Autodesk Fusion 360 part; units mm, degrees
(part 2 of 3)
sketch "Sketch29" plane through (1010, 0, 0) normal (1, 0, 0) x (0, 1, 0)
  circle A0 centre (-195, 872.5) radius 13
  circle A1 centre (-195, 872.5) radius 7.5
  line L0 (-180, 857.5) -> (-210, 857.5)
  line L1 (-210, 857.5) -> (-210, 887.5)
  line L2 (-210, 887.5) -> (-180, 887.5)
  line L3 (-180, 887.5) -> (-180, 857.5)
  line L4 (-180, 857.5) -> (-210, 887.5) construction
  line L5 (-210, 857.5) -> (-180, 887.5) construction
  line L6 (-208, 885.5) -> (-182, 885.5)
  line L7 (-182, 885.5) -> (-182, 859.5)
  line L8 (-182, 859.5) -> (-208, 859.5)
  line L9 (-208, 859.5) -> (-208, 885.5)
  point P0 (-195, 872.5)
  dimension "d267" = 30
  dimension "d268" = 2
  dimension "d269" = 2
  dimension "d270" = 2
  constraint horizontal L0
  constraint perpendicular L0 L1
  constraint parallel L0 L2
  constraint parallel L1 L3
  constraint coincident L4 P0
  constraint coincident L5 P0
  constraint coincident P0 A0.centre
  constraint horizontal L6
  constraint vertical L7
  constraint horizontal L8
  constraint vertical L9
  constraint coincident L4 L7.end
  constraint coincident L4 L6.start
  measures "d267" distance of L0.end L1.end
  measures "d268" distance of L2 L6
  measures "d269" distance of L0 L8
  measures "d270" distance of L3 L7
extrude "Extrude17" add sketch "Sketch29" against normal blind 35 contours L0 L1 L2 L3 bodies 9 in component "bin case (1)"
extrude "Extrude18" cut 1 faces at (1023.3333, -530, 856.6667) along direction (0, 1, 0) blind 30 on bodies 9 bodies 9 in component "bin case (1)"
sketch "Sketch30" plane through (1015, 0, 0) normal (-1, 0, 0) x (0, -1, 0)
  line L0 (500, 840) -> (500, 865)
  line L1 (500, 865) -> (180, 865)
  line L2 (180, 865) -> (180, 875)
  line L3 (180, 875) -> (155, 875)
  line L4 (155, 875) -> (155, 825)
  line L5 (155, 825) -> (180, 825)
  line L6 (180, 825) -> (180, 840)
  line L7 (180, 840) -> (500, 840)
extrude "Extrude19" cut 1 faces at (1023.3333, -500, 856.6667) along direction (0, 1, 0) blind 250 on bodies 9 bodies 9 in component "bin case (1)"
sketch "Sketch31" plane through (0, -180, 0) normal (0, -1, 0) x (1, 0, 0)
  line L0 (1010, 887.5) -> (1010, 875)
  line L1 (1010, 875) -> (1015, 875)
  line L2 (1015, 875) -> (1015, 865)
  line L3 (1015, 865) -> (1040, 865)
  line L4 (1040, 865) -> (1040, 900)
  line L5 (1040, 900) -> (-460, 900)
  line L6 (-460, 900) -> (-485, 900)
  line L7 (-485, 900) -> (-485, 875)
  line L8 (-485, 875) -> (-485, 825)
  line L9 (-485, 825) -> (-486, 825)
  line L10 (-486, 825) -> (-519.6212, 807.8463)
  arc A0 (-519.6212, 807.8463) -> (-535, 775.0001) centre (-534.95, 795) ccw
  line L11 (-535, 775.0001) -> (-535, 775)
  line L12 (-535, 775) -> (-534.9999, 775.0001)
  arc A1 (-534.9999, 775.0001) -> (-518.7278, 783.3022) centre (-534.95, 795) ccw
  line L13 (-518.7278, 783.3022) -> (-486, 800)
  line L14 (-486, 800) -> (-485, 800)
  line L15 (-485, 800) -> (-485, 0)
  line L16 (-485, 0) -> (1040, 0)
  line L17 (1040, 0) -> (1040, 800)
  line L18 (1040, 800) -> (1220, 800)
  line L19 (1220, 800) -> (1248.0189, 784.434)
  arc A2 (1248.0189, 784.434) -> (1250.0621, 808.2988) centre (1265, 795) ccw
  line L20 (1250.0621, 808.2988) -> (1220, 825)
  line L21 (1220, 825) -> (1040, 825)
  line L22 (1040, 825) -> (1040, 840)
  line L23 (1040, 840) -> (1015, 840)
  line L24 (1015, 840) -> (1015, 825)
  line L25 (1015, 825) -> (-460, 825)
  line L26 (-460, 825) -> (-460, 875)
  line L27 (-460, 875) -> (975, 875)
  line L28 (975, 875) -> (975, 887.5)
  line L29 (975, 887.5) -> (1010, 887.5)
  line L30 (-460, 800) -> (265, 800)
  line L31 (265, 800) -> (265, 25)
  line L32 (265, 25) -> (-460, 25)
  line L33 (-460, 25) -> (-460, 800)
  line L34 (290, 800) -> (1015, 800)
  line L35 (1015, 800) -> (1015, 25)
  line L36 (1015, 25) -> (290, 25)
  line L37 (290, 25) -> (290, 800)
  line L38 (1040, 900) -> (1015, 900)
  line L39 (1015, 900) -> (1015, 885)
  line L40 (1015, 885) -> (1040, 885)
  line L41 (1040, 885) -> (1040, 900)
  constraint horizontal L38
  constraint vertical L39
  constraint horizontal L40
  constraint vertical L41
  constraint coincident L4.end L5.start
extrude "Extrude20" add sketch "Sketch31" along normal blind 40 contours L4 L5 L38 L39 L40 L41 bodies 9 in component "bin case (1)"
sketch "Sketch32" plane through (0, -220, 0) normal (0, -1, 0) x (1, 0, 0)
  line L0 (1040, 885) -> (1040, 900)
  line L1 (1040, 900) -> (1015, 900)
  line L2 (1015, 900) -> (1015, 885)
  line L3 (1015, 885) -> (1040, 885)
  line L4 (1015, 900) -> (1040, 900)
  line L5 (1040, 900) -> (1040, 875)
  line L6 (1040, 875) -> (1015, 875)
  line L7 (1015, 875) -> (1015, 900)
  dimension "d283" = 25
  constraint horizontal L4
  constraint vertical L5
  constraint horizontal L6
  constraint vertical L7
  constraint coincident L1.end L2.start
  measures "d283" distance of L1.end L6.end
extrude "Extrude21" add sketch "Sketch32" along normal blind 290 bodies 9 in component "bin case (1)"
extrude "Extrude22" cut 1 faces at (1023.3333, -250, 856.6667) along direction (0, 1, 0) blind 10 on bodies 9 bodies 9 in component "bin case (1)"
sketch "Sketch33" plane through (0, 0, 865) normal (0, 0, 1) x (-1, 0, 0)
  line L0 (-1015, 240) -> (-1040, 240)
  line L1 (-1040, 240) -> (-1040, 180)
  line L2 (-1040, 180) -> (-1015, 180)
  line L3 (-1015, 180) -> (-1015, 240)
  line L4 (-1015, 240) -> (-1040, 240)
  line L5 (-1040, 240) -> (-1040, 215)
  line L6 (-1040, 215) -> (-1015, 215)
  line L7 (-1015, 215) -> (-1015, 240)
  constraint horizontal L4
  constraint vertical L5
  constraint horizontal L6
  constraint vertical L7
  constraint coincident L1 L5.end
  constraint coincident L0.start L3.end
extrude "Extrude23" add sketch "Sketch33" along normal blind 20 contours L0 L1 L3 L4 L5 L6 L7 bodies 9 in component "bin case (1)"
sketch "Sketch34" plane through (1015, 0, 0) normal (-1, 0, 0) x (0, -1, 0)
  line L0 (240, 840) -> (240, 875)
  line L1 (240, 875) -> (510, 875)
  line L2 (510, 875) -> (510, 900)
  line L3 (510, 900) -> (180, 900)
  line L4 (180, 900) -> (180, 885)
  line L5 (180, 885) -> (215, 885)
  line L6 (215, 885) -> (215, 865)
  line L7 (215, 865) -> (180, 865)
  line L8 (180, 865) -> (180, 875)
  line L9 (180, 875) -> (155, 875)
  line L10 (155, 875) -> (155, 825)
  line L11 (155, 825) -> (180, 825)
  line L12 (180, 825) -> (180, 840)
  line L13 (180, 840) -> (240, 840)
  circle A0 centre (545, 872.5) radius 27.5
  line L14 (510, 900) -> (545, 882.5)
  line L15 (510, 875) -> (545, 857.5)
  line L16 (545, 857.5) -> (545, 882.5)
  circle A1 centre (545, 872.5) radius 15
  constraint coincident L2.end L3.start
  constraint coincident L1.end L2.start
  constraint parallel L14 L15
  constraint vertical L16
  constraint concentric A0 A1
  constraint coincident L15.end A1
extrude "Extrude24" add sketch "Sketch34" against normal blind 25 contours L2 A0 L14 L15 | A0 L14 L15 A1 | L14 L15 L16 A1 | L15 A1 | L14 L16 A1 picked at (527.3778, 887.7148) bodies 9 in component "bin case (1)"
sketch "Sketch35" plane through (1040, 0, 0) normal (1, 0, 0) x (0, 1, 0)
  line L0 (-240, 875) -> (-240, 840)
  line L1 (-240, 840) -> (-180, 840)
  line L2 (-180, 840) -> (-180, 825)
  line L3 (-180, 825) -> (-155, 825)
  line L4 (-155, 825) -> (-155, 900)
  line L5 (-155, 900) -> (-510, 900)
  line L6 (-510, 900) -> (-538.2297, 885.8852)
  arc A0 (-538.2297, 885.8852) -> (-533, 863.5) centre (-545, 872.5) ccw
  line L7 (-533, 863.5) -> (-510, 875)
  line L8 (-510, 875) -> (-240, 875)
  line L9 (-215, 865) -> (-215, 885)
  line L10 (-215, 885) -> (-180, 885)
  line L11 (-180, 885) -> (-180, 865)
  line L12 (-180, 865) -> (-215, 865)
  circle A1 centre (-545, 872.5) radius 15
  constraint concentric A0 A1
extrude "Extrude25" add sketch "Sketch35" along normal blind 5 contours A0 A1 bodies 9 in component "bin case (1)"
ref_plane "WorkPlane2" through (1245, -360.0396, 862.5) normal (1, 0, 0) x (0, 1, 0)
sketch "Sketch36" plane through (1245, 0, 0) normal (1, 0, 0) x (0, 1, 0)
  circle A0 centre (-545, 872.5) radius 27.5
  circle A1 centre (-195, 872.5) radius 27.5
  circle A2 centre (-545, 872.5) radius 15
  circle A3 centre (-195, 872.5) radius 15
  dimension "d296" = 30
  dimension "d297" = 30
  constraint concentric A0 A2
  constraint concentric A1 A3
  measures "d296" diameter of A2
  measures "d297" diameter of A3
extrude "Extrude6''" add sketch "Sketch36" along normal blind 5 separate body contours A2 | A3 makes body 21 at (1245, -541.6161, 875.3166) makes body 22 at (1245, -199.4126, 875.9009)
copy_body "CutPasteBodies4" bodies 22 21 removing the originals makes body 23 makes body 24 in component "bin case (1)"
sketch "Sketch37" plane through (1250, 0, 0) normal (1, 0, 0) x (0, 1, 0)
  circle A0 centre (-545, 872.5) radius 15
  line L0 (-510.0236, 899.9783) -> (-220.0236, 899.9783)
  line L1 (-220.0236, 899.9783) -> (-220.0236, 874.9783)
  line L2 (-220.0236, 874.9783) -> (-510.0236, 874.9783)
  line L3 (-510.0236, 874.9783) -> (-510.0236, 899.9783)
  line L4 (-510.0236, 874.9783) -> (-545, 857.5)
  line L5 (-510.0236, 899.9783) -> (-545, 882.5)
  line L6 (-545, 882.5) -> (-545, 857.5)
  line L7 (-220.0236, 899.9783) -> (-195, 887.6217)
  line L8 (-220.0236, 874.9783) -> (-195, 862.6217)
  line L9 (-195, 862.6217) -> (-195, 887.6217)
  circle A1 centre (-195, 872.5) radius 15
  circle A2 centre (-195, 872.5) radius 15
  dimension "d300" = 290
  dimension "d301" = 25
  dimension "d302" = 30
  constraint horizontal L0
  constraint vertical L1
  constraint horizontal L2
  constraint vertical L3
  constraint coincident A0 L4.end
  constraint parallel L4 L5
  constraint perpendicular L2 L6
  constraint parallel L7 L8
  constraint perpendicular L2 L9
  constraint coincident L9 A1.centre
  constraint concentric A1 A2
  measures "d300" distance of L0.start L0.end
  measures "d301" distance of L0 L2
  measures "d302" diameter of A1
extrude "Extrude26" add sketch "Sketch37" along normal blind 25 bodies 23 24 in component "bin case (1)"
sketch "Sketch38" plane through (0, 0, 874.9783) normal (0, 0, -1) x (1, 0, 0)
  line L0 (1250, 510.0236) -> (1250, 220.0236)
  line L1 (1250, 220.0236) -> (1275, 220.0236)
  line L2 (1275, 220.0236) -> (1275, 510.0236)
  line L3 (1275, 510.0236) -> (1250, 510.0236)
  line L4 (1250, 220.0236) -> (1275, 220.0236)
  line L5 (1275, 220.0236) -> (1275, 245.0236)
  line L6 (1275, 245.0236) -> (1250, 245.0236)
  line L7 (1250, 245.0236) -> (1250, 220.0236)
  dimension "d305" = 25
  constraint horizontal L4
  constraint vertical L5
  constraint horizontal L6
  constraint vertical L7
  constraint coincident L2 L5.end
  constraint coincident L0.end L1.start
  measures "d305" distance of L4 L6
extrude "Extrude27" add sketch "Sketch38" along normal blind 75 contours L0 L1 L2 L4 L5 L6 L7 bodies 23 in component "bin case (1)"
sketch "Sketch39" plane through (1250, 0, 0) normal (-1, 0, 0) x (0, -1, 0)
  arc A0 (209.7761, 869.9181) -> (195, 887.5) centre (195, 872.5) ccw
  line L0 (209.7761, 869.9181) -> (220.0236, 874.9783)
  line L1 (220.0236, 874.9783) -> (220.0236, 799.9783)
  line L2 (220.0236, 799.9783) -> (245.0236, 799.9783)
  line L3 (245.0236, 799.9783) -> (245.0236, 874.9783)
  line L4 (245.0236, 874.9783) -> (510.0236, 874.9783)
  line L5 (510.0236, 874.9783) -> (533.0041, 863.4946)
  arc A1 (538.2278, 885.8842) -> (533.0041, 863.4946) centre (545, 872.5) ccw
  line L6 (538.2278, 885.8842) -> (510.0236, 899.9783)
  line L7 (510.0236, 899.9783) -> (220.0236, 899.9783)
  line L8 (220.0236, 899.9783) -> (195, 887.6217)
  line L9 (195, 887.6217) -> (195, 887.5)
  line L10 (245.0236, 799.9783) -> (220.0236, 799.9783)
  line L11 (220.0236, 799.9783) -> (220.0236, 824.9783)
  line L12 (220.0236, 824.9783) -> (245.0236, 824.9783)
  line L13 (245.0236, 824.9783) -> (245.0236, 799.9783)
  dimension "d308" = 25
  constraint horizontal L10
  constraint vertical L11
  constraint horizontal L12
  constraint vertical L13
  constraint coincident L2.end L3.start
  measures "d308" distance of L2.end L12.end
extrude "Extrude28" add sketch "Sketch39" along normal blind 235 contours L1 L2 L3 L10 L11 L12 L13 bodies 23 in component "bin case (1)"
sketch "Sketch40" plane through (0, -180, 0) normal (0, -1, 0) x (1, 0, 0)
  line L0 (1015, 885) -> (1015, 900)
  line L1 (1015, 900) -> (-460, 900)
  line L2 (-460, 900) -> (-485, 900)
  line L3 (-485, 900) -> (-485, 875)
  line L4 (-485, 875) -> (-485, 825)
  line L5 (-485, 825) -> (-486, 825)
  line L6 (-486, 825) -> (-519.6212, 807.8463)
  arc A0 (-519.6212, 807.8463) -> (-535, 775.0001) centre (-534.95, 795) ccw
  line L7 (-535, 775.0001) -> (-535, 775)
  line L8 (-535, 775) -> (-534.9999, 775.0001)
  arc A1 (-534.9999, 775.0001) -> (-518.7278, 783.3022) centre (-534.95, 795) ccw
  line L9 (-518.7278, 783.3022) -> (-486, 800)
  line L10 (-486, 800) -> (-485, 800)
  line L11 (-485, 800) -> (-485, 0)
  line L12 (-485, 0) -> (1040, 0)
  line L13 (1040, 0) -> (1040, 800)
  line L14 (1040, 800) -> (1220, 800)
  line L15 (1220, 800) -> (1248.0189, 784.434)
  arc A2 (1248.0189, 784.434) -> (1250.0621, 808.2988) centre (1265, 795) ccw
  line L16 (1250.0621, 808.2988) -> (1220, 825)
  line L17 (1220, 825) -> (1040, 825)
  line L18 (1040, 825) -> (1040, 840)
  line L19 (1040, 840) -> (1015, 840)
  line L20 (1015, 840) -> (1015, 825)
  line L21 (1015, 825) -> (-460, 825)
  line L22 (-460, 825) -> (-460, 875)
  line L23 (-460, 875) -> (975, 875)
  line L24 (975, 875) -> (975, 887.5)
  line L25 (975, 887.5) -> (1010, 887.5)
  line L26 (1010, 887.5) -> (1010, 875)
  line L27 (1010, 875) -> (1015, 875)
  line L28 (1015, 875) -> (1015, 865)
  line L29 (1015, 865) -> (1040, 865)
  line L30 (1040, 865) -> (1040, 885)
  line L31 (1040, 885) -> (1015, 885)
  line L32 (-460, 800) -> (265, 800)
  line L33 (265, 800) -> (265, 25)
  line L34 (265, 25) -> (-460, 25)
  line L35 (-460, 25) -> (-460, 800)
  line L36 (290, 800) -> (1015, 800)
  line L37 (1015, 800) -> (1015, 25)
  line L38 (1015, 25) -> (290, 25)
  line L39 (290, 25) -> (290, 800)
  line L40 (1015, 825) -> (1040, 825)
  line L41 (1040, 825) -> (1040, 800)
  line L42 (1040, 800) -> (1015, 800)
  line L43 (1015, 800) -> (1015, 825)
  constraint horizontal L40
  constraint vertical L41
  constraint horizontal L42
  constraint vertical L43
  constraint coincident L13.end L14.start
  constraint coincident L20.end L21.start
extrude "Extrude29" add sketch "Sketch40" along normal blind 65 contours L40 L41 L42 L43 bodies 9 23 in component "bin case (1)"
sketch "Sketch41" plane through (1015, 0, 0) normal (-1, 0, 0) x (0, -1, 0)
  line L0 (240, 840) -> (240, 875)
  line L1 (240, 875) -> (510, 875)
  line L2 (510, 875) -> (533, 863.5)
  arc A0 (533, 863.5) -> (538.2297, 885.8852) centre (545, 872.5) ccw
  line L3 (538.2297, 885.8852) -> (510, 900)
  line L4 (510, 900) -> (180, 900)
  line L5 (180, 900) -> (180, 885)
  line L6 (180, 885) -> (215, 885)
  line L7 (215, 885) -> (215, 865)
  line L8 (215, 865) -> (180, 865)
  line L9 (180, 865) -> (180, 875)
  line L10 (180, 875) -> (155, 875)
  line L11 (155, 875) -> (155, 825)
  line L12 (155, 825) -> (180, 825)
  line L13 (180, 825) -> (180, 840)
  line L14 (180, 840) -> (240, 840)
sketch "Sketch42" plane through (1015, 0, 0) normal (-1, 0, 0) x (0, -1, 0)
  line L0 (220.0236, 800) -> (220.0236, 799.9783)
  line L1 (220.0236, 799.9783) -> (245.0236, 799.9783)
  line L2 (245.0236, 799.9783) -> (245.0236, 824.9783)
  line L3 (245.0236, 824.9783) -> (245, 824.9783)
  line L4 (245, 824.9783) -> (245, 825)
  line L5 (245, 825) -> (180, 825)
  line L6 (180, 825) -> (180, 800)
  line L7 (180, 800) -> (220.0236, 800)
  line L8 (245.0236, 799.9783) -> (220, 799.9783)
  line L9 (220, 799.9783) -> (220, 825)
  line L10 (220, 825) -> (245.0236, 825)
  line L11 (245.0236, 825) -> (245.0236, 799.9783)
  constraint horizontal L8
  constraint vertical L9
  constraint horizontal L10
  constraint vertical L11
  constraint coincident L5 L9.end
  constraint coincident L1.end L2.start
extrude "Extrude30" add sketch "Sketch42" along normal blind 25 contours L0 L1 L2 L3 L4 L5 L7 L8 L9 L10 L11 bodies 9 in component "bin case (1)"
sketch "Sketch43" plane through (0, 0, 825) normal (0, 0, 1) x (-1, 0, 0)
  line L0 (-1040, 180) -> (-1015, 180)
  line L1 (-1015, 180) -> (-1015, 220)
  line L2 (-1015, 220) -> (-990, 220)
  line L3 (-990, 220) -> (-990, 245)
  line L4 (-990, 245) -> (-1040, 245)
  line L5 (-1040, 245) -> (-1040, 180)
  line L6 (-990, 220) -> (-1015, 220)
  line L7 (-1015, 220) -> (-1015, 245)
  line L8 (-1015, 245) -> (-990, 245)
  line L9 (-990, 245) -> (-990, 220)
  constraint horizontal L6
  constraint vertical L7
  constraint horizontal L8
  constraint vertical L9
  constraint midpoint L4 L7.end
  constraint coincident L2.end L3.start
extrude "Extrude31" add sketch "Sketch43" along normal blind 250 contours L2 L3 L4 L6 L7 L8 L9 bodies 9 in component "bin case (1)"
sketch "Sketch44" plane through (0, -180, 0) normal (0, -1, 0) x (1, 0, 0)
  line L0 (1040, 825) -> (1040, 800)
  line L1 (1040, 800) -> (1220, 800)
  line L2 (1220, 800) -> (1248.0189, 784.434)
  arc A0 (1248.0189, 784.434) -> (1250.0621, 808.2988) centre (1265, 795) ccw
  line L3 (1250.0621, 808.2988) -> (1220, 825)
  line L4 (1220, 825) -> (1040, 825)
  line L5 (1140, 825) -> (1165, 825)
  line L6 (1165, 825) -> (1165, 800)
  line L7 (1165, 800) -> (1140, 800)
  line L8 (1140, 800) -> (1140, 825)
  dimension "d322" = 25
  dimension "d323" = 100
  constraint horizontal L5
  constraint vertical L6
  constraint horizontal L7
  constraint vertical L8
  constraint coincident L1 L6.end
  constraint coincident L4 L5.start
  measures "d322" distance of L6 L8
  measures "d323" distance of L0 L8
extrude "Extrude32" add sketch "Sketch44" along normal blind 45 contours L1 L4 L5 L6 L7 L8 bodies 9 in component "bin case (1)"
sketch "Sketch45" plane through (1015, 0, 0) normal (-1, 0, 0) x (0, -1, 0)
  line L0 (155, 25) -> (180, 25)
  line L1 (180, 25) -> (180, 800)
  line L2 (180, 800) -> (155, 800)
  line L3 (155, 800) -> (155, 25)
  line L4 (220, 800) -> (180, 765)
  line L5 (245, 800) -> (180, 743.125)
  line L6 (180, 765) -> (180, 743.125)
  line L7 (220, 800) -> (245, 800)
  constraint coincident L1 L4.end
  constraint coincident L1 L5.end
  constraint parallel L4 L5
  constraint perpendicular L1 L7
extrude "Extrude33" add sketch "Sketch45" against normal blind 25 contours L1 L4 L5 L6 L7 bodies 9 in component "bin case (1)"
sketch "Sketch46" plane through (0, -245, 0) normal (0, -1, 0) x (1, 0, 0)
  line L0 (990, 824.9783) -> (1040, 824.9783)
  line L1 (1040, 824.9783) -> (1040, 825)
  line L2 (1040, 825) -> (1015, 825)
  line L3 (1015, 825) -> (1015, 875)
  line L4 (1015, 875) -> (1015, 900)
  line L5 (1015, 900) -> (1015, 1075)
  line L6 (1015, 1075) -> (990, 1075)
  line L7 (990, 1075) -> (990, 824.9783)
  line L8 (990, 1075) -> (1015, 1075)
  line L9 (1015, 1075) -> (1015, 1050)
  line L10 (1015, 1050) -> (990, 1050)
  line L11 (990, 1050) -> (990, 1075)
  dimension "d328" = 25
  constraint horizontal L8
  constraint vertical L9
  constraint horizontal L10
  constraint vertical L11
  constraint coincident L6.end L7.start
  measures "d328" distance of L6.end L10.end
extrude "Extrude34" add sketch "Sketch46" along normal blind 200 contours L5 L6 L7 L8 L9 L10 L11 bodies 9 in component "bin case (1)"
sketch "Sketch47" plane through (1015, 0, 0) normal (1, 0, 0) x (0, 1, 0)
  line L0 (-245, 900) -> (-220, 900)
  line L1 (-220, 900) -> (-220, 1075)
  line L2 (-220, 1075) -> (-445, 1075)
  line L3 (-445, 1075) -> (-445, 1050)
  line L4 (-445, 1050) -> (-245, 1050)
  line L5 (-245, 1050) -> (-245, 900)
  line L6 (-445, 1075) -> (-345, 1075)
  line L7 (-345, 1075) -> (-345, 1025)
  line L8 (-345, 1025) -> (-445, 1025)
  line L9 (-445, 1025) -> (-445, 1075)
  dimension "d331" = 50
  constraint horizontal L6
  constraint vertical L7
  constraint horizontal L8
  constraint vertical L9
  constraint coincident L2.end L3.start
  measures "d331" distance of L2.end L8.end
extrude "Extrude1'''''''''" add sketch "Sketch47" along normal blind 250 separate body contours L4 L7 L8 L9 | L2 L3 L4 L6 L7 L9 makes body 25 in component "cam"
sketch "Sketch48" plane through (0, 0, 1025) normal (0, 0, -1) x (1, 0, 0)
  line L0 (1015, 445) -> (1015, 345)
  line L1 (1015, 345) -> (1265, 345)
  line L2 (1265, 345) -> (1265, 445)
  line L3 (1265, 445) -> (1015, 445)
  circle A0 centre (1140, 395) radius 10
  dimension "d336" = 20
  dimension "d337" = 50
  dimension "d338" = 125
  measures "d336" diameter of A0
  measures "d337" distance of L3 A0.centre
  measures "d338" distance of L0 A0.centre
extrude "Extrude2''''''''" add sketch "Sketch48" along normal blind 10 contours A0 bodies 25 in component "cam"
sketch "Sketch49" plane through (0, 0, 1015) normal (0, 0, -1) x (1, 0, 0)
  circle A0 centre (1140, 395) radius 10
  circle A1 centre (1140, 395) radius 5
  constraint concentric A0 A1
extrude "Extrude3''''" add sketch "Sketch49" along normal blind 5 contours A1 bodies 25 in component "cam"
sketch "Sketch50" plane through (0, 0, 900) normal (0, 0, 1) x (-1, 0, 0)
  line L0 (225, 97.8741) -> (185, 155)
  line L1 (185, 155) -> (225, 155)
  line L2 (225, 155) -> (225, 97.8741)
  line L3 (250, 62.1704) -> (250, 155)
  line L4 (250, 155) -> (485, 155)
  line L5 (485, 155) -> (485, 180)
  line L6 (485, 180) -> (460, 180)
  line L7 (460, 180) -> (-1015, 180)
  line L8 (-1015, 180) -> (-1015, 220)
  line L9 (-1015, 220) -> (-1015, 245)
  line L10 (-1015, 245) -> (-1015, 510)
  line L11 (-1015, 510) -> (-1040, 510)
  line L12 (-1040, 510) -> (-1040, 155)
  line L13 (-1040, 155) -> (160, 155)
  line L14 (160, 155) -> (451.3094, -268.9154)
  line L15 (451.3094, -268.9154) -> (471.7882, -254.576)
  line L16 (471.7882, -254.576) -> (250, 62.1704)
  line L17 (-265.0737, 155) -> (-290, 155)
  line L18 (-290, 155) -> (-290, 180)
  line L19 (-290, 180) -> (-265.0737, 180)
  line L20 (-265.0737, 180) -> (-265.0737, 155)
  line L21 (-640, 155) -> (-665, 155)
  line L22 (-665, 155) -> (-665, 180)
  line L23 (-665, 180) -> (-640, 180)
  line L24 (-640, 180) -> (-640, 155)
  line L25 (-1015, 155) -> (-1040, 155)
  line L26 (-1040, 155) -> (-1040, 180)
  line L27 (-1040, 180) -> (-1015, 180)
  line L28 (-1015, 180) -> (-1015, 155)
  constraint horizontal L17
  constraint vertical L18
  constraint horizontal L19
  constraint vertical L20
  constraint coincident L7 L18.end
  constraint coincident L13 L17.start
  constraint horizontal L21
  constraint vertical L22
  constraint horizontal L23
  constraint vertical L24
  constraint coincident L7 L22.end
  constraint coincident L13 L21.start
  constraint horizontal L25
  constraint vertical L26
  constraint horizontal L27
  constraint vertical L28
  constraint coincident L12 L26.end
  constraint coincident L13 L25.start
sketch "Sketch51" plane through (0, -155, 0) normal (0, 1, 0) x (-1, 0, 0)
  line L0 (250, 900) -> (250, 875)
  line L1 (250, 875) -> (460, 875)
  line L2 (460, 875) -> (460, 825)
  line L3 (460, 825) -> (-1015, 825)
  line L4 (-1015, 825) -> (-1015, 875)
  line L5 (-1015, 875) -> (160, 875)
  line L6 (160, 875) -> (160, 900)
  line L7 (160, 900) -> (-1040, 900)
  line L8 (-1040, 900) -> (-1040, 825)
  line L9 (-1040, 825) -> (-1220, 825)
  line L10 (-1220, 825) -> (-1250.0621, 808.2988)
  arc A0 (-1248.0189, 784.434) -> (-1250.0621, 808.2988) centre (-1265, 795) ccw
  line L11 (-1248.0189, 784.434) -> (-1220, 800)
  line L12 (-1220, 800) -> (-1040, 800)
  line L13 (-1040, 800) -> (-1040, 25)
  line L14 (-1040, 25) -> (-1015, 25)
  line L15 (-1015, 25) -> (-1015, 800)
  line L16 (-1015, 800) -> (-290, 800)
  line L17 (-290, 800) -> (-290, 25)
  line L18 (-290, 25) -> (-265, 25)
  line L19 (-265, 25) -> (-265, 800)
  line L20 (-265, 800) -> (460, 800)
  line L21 (460, 800) -> (460, 25)
  line L22 (460, 25) -> (485, 25)
  line L23 (485, 25) -> (485, 800)
  line L24 (485, 800) -> (486, 800)
  line L25 (486, 800) -> (518.7278, 783.3022)
  arc A1 (519.6212, 807.8463) -> (518.7278, 783.3022) centre (534.95, 795) ccw
  line L26 (519.6212, 807.8463) -> (486, 825)
  line L27 (486, 825) -> (485, 825)
  line L28 (485, 825) -> (485, 875)
  line L29 (485, 875) -> (485, 900)
  line L30 (485, 900) -> (250, 900)
  line L31 (-1015, 875) -> (-990, 875)
  line L32 (-990, 875) -> (-990, 900)
  line L33 (-990, 900) -> (-1015, 900)
  line L34 (-1015, 900) -> (-1015, 875)
  line L35 (-615, 875) -> (-640, 875)
  line L36 (-640, 875) -> (-640, 900)
  line L37 (-640, 900) -> (-615, 900)
  line L38 (-615, 900) -> (-615, 875)
  line L39 (-240, 875) -> (-265, 875)
  line L40 (-265, 875) -> (-265, 900)
  line L41 (-265, 900) -> (-240, 900)
  line L42 (-240, 900) -> (-240, 875)
  dimension "d343" = 25
  dimension "d344" = 25
  dimension "d345" = 25
  constraint horizontal L31
  constraint vertical L32
  constraint horizontal L33
  constraint vertical L34
  constraint coincident L7 L32.end
  constraint coincident L4.end L5.start
  constraint horizontal L35
  constraint vertical L36
  constraint horizontal L37
  constraint vertical L38
  constraint coincident L7 L36.end
  constraint coincident L5 L35.start
  constraint horizontal L39
  constraint vertical L40
  constraint horizontal L41
  constraint vertical L42
  constraint coincident L7 L40.end
  constraint coincident L5 L39.start
  measures "d343" distance of L32 L34
  measures "d344" distance of L36 L38
  measures "d345" distance of L40 L42
sketch "Sketch52" plane through (0, 0, 825) normal (0, 0, 1) x (-1, 0, 0)
  line L0 (-1015, 180) -> (-1015, 155)
  line L1 (-1015, 155) -> (460, 155)
  line L2 (460, 155) -> (460, 180)
  line L3 (460, 180) -> (-1015, 180)
  circle A0 centre (-965, 167.5) radius 12.5
  circle A1 centre (-590, 167.5) radius 12.5
  circle A2 centre (-215, 167.5) radius 12.5
  dimension "d346" = 50
  dimension "d349" = 750
  dimension "d350" = 0
  constraint tangent L1 A0
  measures "d346" distance of L0 A0.centre
extrude "Extrude35" add sketch "Sketch52" along normal blind 10 contours A0 | A1 | A2 bodies 9 in component "bin case (1)"
sketch "Sketch53" plane through (0, 0, 835) normal (0, 0, 1) x (-1, 0, 0)
  circle A0 centre (-215, 167.5) radius 12.5
  circle A1 centre (-215, 167.5) radius 17.5
  dimension "d353" = 35
  constraint concentric A0 A1
  measures "d353" diameter of A1
extrude "Extrude1''''''''''" add sketch "Sketch53" along normal blind 40 separate body contours A0 | A1 makes body 26 in component "paddle1"
sketch "Sketch54" plane through (0, 0, 875) normal (0, 0, 1) x (-1, 0, 0)
  circle A0 centre (-215, 167.5) radius 17.5
  circle A1 centre (-215, 167.5) radius 10
  line L0 (-215, 157.5) -> (-215, 177.5)
  line L1 (-215, 177.5) -> (135, 177.5)
  line L2 (135, 177.5) -> (135, 157.5)
  line L3 (135, 157.5) -> (-215, 157.5)
  dimension "d356" = 20
  dimension "d357" = 350
  constraint concentric A0 A1
  constraint perpendicular L0 L1
  constraint parallel L0 L2
  constraint parallel L1 L3
  constraint coincident A1 L0.end
  constraint vertical L0
  constraint coincident A1 L0.start
  measures "d356" diameter of A1
  measures "d357" distance of L0.start L2.end
extrude "Extrude7'" add sketch "Sketch54" against normal blind 40 separate body contours A0 L1 L2 L3 makes body 27
copy_body "CutPasteBodies1''" bodies 27 removing the originals makes body 28 in component "paddle1"
sketch "Sketch55" plane through (0, 0, 825) normal (0, 0, 1) x (-1, 0, 0)
  line L0 (-640.0675, -475) -> (-640.0675, -100)
  line L1 (-640.0675, -100) -> (-290.0675, -100)
  line L2 (-290.0675, -100) -> (-290.0675, -475)
  line L3 (-290.0675, -475) -> (-265.0675, -475)
  line L4 (-265.0675, -475) -> (-265.0675, -100)
  line L5 (-265.0675, -100) -> (84.9325, -100)
  line L6 (84.9325, -100) -> (84.9325, -475)
  line L7 (84.9325, -475) -> (109.9325, -475)
  line L8 (109.9325, -475) -> (109.9325, -100)
  line L9 (109.9325, -100) -> (459.9325, -100)
  line L10 (459.9325, -100) -> (459.9325, -475)
  line L11 (459.9325, -475) -> (484.9325, -475)
  line L12 (484.9325, -475) -> (484.9325, -75)
  line L13 (484.9325, -75) -> (-1220.0675, -75)
  line L14 (-1220.0675, -75) -> (-1220.0675, -100)
  line L15 (-1220.0675, -100) -> (-1040.0675, -100)
  line L16 (-1040.0675, -100) -> (-1040.0675, -475)
  line L17 (-1040.0675, -475) -> (-1015.0675, -475)
  line L18 (-1015.0675, -475) -> (-1015.0675, -100)
  line L19 (-1015.0675, -100) -> (-665.0675, -100)
  line L20 (-665.0675, -100) -> (-665.0675, -475)
  line L21 (-665.0675, -475) -> (-640.0675, -475)
  line L22 (-1005.0675, -110) -> (-675.0675, -110)
  line L23 (-675.0675, -110) -> (-675.0675, -440)
  line L24 (-675.0675, -440) -> (-1005.0675, -440)
  line L25 (-1005.0675, -440) -> (-1005.0675, -110)
  line L26 (-1015.0675, -100) -> (-665.0675, -100)
  line L27 (-665.0675, -100) -> (-665.0675, -450)
  line L28 (-665.0675, -450) -> (-1015.0675, -450)
  line L29 (-1015.0675, -450) -> (-1015.0675, -100)
  dimension "d378" = 10
  dimension "d379" = 10
  dimension "d380" = 10
  dimension "d381" = 330
  dimension "d382" = 10
  constraint horizontal L22
  constraint vertical L23
  constraint horizontal L24
  constraint vertical L25
  constraint horizontal L26
  constraint vertical L27
  constraint horizontal L28
  constraint vertical L29
  constraint coincident L20 L27.end
  constraint coincident L18.end L19.start
  measures "d378" distance of L19 L22
  measures "d379" distance of L20 L23
  measures "d380" distance of L18 L25
  measures "d381" distance of L22 L24
  measures "d382" distance of L24 L28
sketch "Sketch56" plane through (0, 0, 25) normal (0, 0, 1) x (-1, 0, 0)
  line L0 (-665.0675, -350) -> (-665.0675, -450)
  line L1 (-665.0675, -450) -> (-640.0675, -450)
  line L2 (-640.0675, -450) -> (-640.0675, -350)
  line L3 (-640.0675, -350) -> (-290.0675, -350)
  line L4 (-290.0675, -350) -> (-290.0675, -450)
  line L5 (-290.0675, -450) -> (-265.0675, -450)
  line L6 (-265.0675, -450) -> (-265.0675, -350)
  line L7 (-265.0675, -350) -> (84.9325, -350)
  line L8 (84.9325, -350) -> (84.9325, -450)
  line L9 (84.9325, -450) -> (109.9325, -450)
  line L10 (109.9325, -450) -> (109.9325, -350)
  line L11 (109.9325, -350) -> (459.9325, -350)
  line L12 (459.9325, -350) -> (459.9325, -450)
  line L13 (459.9325, -450) -> (484.9325, -450)
  line L14 (484.9325, -450) -> (484.9325, -100)
  line L15 (484.9325, -100) -> (459.9325, -100)
  line L16 (459.9325, -100) -> (459.9325, -200)
  line L17 (459.9325, -200) -> (109.9325, -200)
  line L18 (109.9325, -200) -> (109.9325, -100)
  line L19 (109.9325, -100) -> (84.9325, -100)
  line L20 (84.9325, -100) -> (84.9325, -200)
  line L21 (84.9325, -200) -> (-265.0675, -200)
  line L22 (-265.0675, -200) -> (-265.0675, -100)
  line L23 (-265.0675, -100) -> (-290.0675, -100)
  line L24 (-290.0675, -100) -> (-290.0675, -200)
  line L25 (-290.0675, -200) -> (-640.0675, -200)
  line L26 (-640.0675, -200) -> (-640.0675, -100)
  line L27 (-640.0675, -100) -> (-665.0675, -100)
  line L28 (-665.0675, -100) -> (-665.0675, -200)
  line L29 (-665.0675, -200) -> (-1015.0675, -200)
  line L30 (-1015.0675, -200) -> (-1015.0675, -100)
  line L31 (-1015.0675, -100) -> (-1040.0675, -100)
  line L32 (-1040.0675, -100) -> (-1040.0675, -450)
  line L33 (-1040.0675, -450) -> (-1015.0675, -450)
  line L34 (-1015.0675, -450) -> (-1015.0675, -350)
  line L35 (-1015.0675, -350) -> (-665.0675, -350)
  line L36 (-640.0675, -325) -> (-640.0675, -225)
  line L37 (-640.0675, -225) -> (-290.0675, -225)
  line L38 (-290.0675, -225) -> (-290.0675, -325)
  line L39 (-290.0675, -325) -> (-640.0675, -325)
  line L40 (-665.0675, -325) -> (-1015.0675, -325)
  line L41 (-1015.0675, -325) -> (-1015.0675, -225)
  line L42 (-1015.0675, -225) -> (-665.0675, -225)
  line L43 (-665.0675, -225) -> (-665.0675, -325)
  line L44 (109.9325, -325) -> (109.9325, -225)
  line L45 (109.9325, -225) -> (459.9325, -225)
  line L46 (459.9325, -225) -> (459.9325, -325)
  line L47 (459.9325, -325) -> (109.9325, -325)
  line L48 (84.9325, -325) -> (-265.0675, -325)
  line L49 (-265.0675, -325) -> (-265.0675, -225)
  line L50 (-265.0675, -225) -> (84.9325, -225)
  line L51 (84.9325, -225) -> (84.9325, -325)
  line L52 (-995.0675, -120) -> (-685.0675, -120)
  line L53 (-685.0675, -120) -> (-685.0675, -430)
  line L54 (-685.0675, -430) -> (-995.0675, -430)
  line L55 (-995.0675, -430) -> (-995.0675, -120)
  line L56 (-1015.0675, -100) -> (-665.0675, -100)
  line L57 (-665.0675, -450) -> (-1015.0675, -450)
  line L58 (-665.0675, -100) -> (-665.0675, -450)
  line L59 (-1015.0675, -450) -> (-1015.0675, -100)
  dimension "d383" = 20
  dimension "d384" = 20
  dimension "d385" = 20
  dimension "d386" = 20
  constraint horizontal L52
  constraint vertical L53
  constraint horizontal L54
  constraint vertical L55
  measures "d383" distance of L52 L56
  measures "d384" distance of L54 L57
  measures "d385" distance of L53 L58
  measures "d386" distance of L55 L59
loft "Loft1" add profiles "Sketch55", "Sketch56" section 1 contours L18 L19 L20 L26 L27 L28 L29 | L22 L23 L24 L25 section 2 contours L35 L53 L54 L55 | L35 L40 L53 L55 | L40 L42 L53 L55 | L29 L42 L53 L55 | L29 L52 L53 L55 separate body makes body 29 in component "bin"
shell "Shell1" thickness 10 removed faces 1 at (781.7342, 216.6667, 825) on bodies 29 in component "bin"
loft "Loft1'" add profiles "Sketch55", "Sketch56" section 1 contours L18 L19 L20 L26 L27 L28 L29 | L22 L23 L24 L25 section 2 contours L35 L53 L54 L55 | L35 L40 L53 L55 | L40 L42 L53 L55 | L29 L42 L53 L55 | L29 L52 L53 L55 separate body makes body 30 in component "bin (1)"
shell "Shell1'" thickness 10 removed faces 1 at (781.7342, 216.6667, 825) on bodies 30 in component "bin (1)"
loft "Loft1''" add profiles "Sketch55", "Sketch56" section 1 contours L18 L19 L20 L26 L27 L28 L29 | L22 L23 L24 L25 section 2 contours L35 L53 L54 L55 | L35 L40 L53 L55 | L40 L42 L53 L55 | L29 L42 L53 L55 | L29 L52 L53 L55 separate body makes body 31 in component "bin (2)"
shell "Shell1''" thickness 10 removed faces 1 at (781.7342, 216.6667, 825) on bodies 31 in component "bin (2)"
loft "Loft1'''" add profiles "Sketch55", "Sketch56" section 1 contours L18 L19 L20 L26 L27 L28 L29 | L22 L23 L24 L25 section 2 contours L35 L53 L54 L55 | L35 L40 L53 L55 | L40 L42 L53 L55 | L29 L42 L53 L55 | L29 L52 L53 L55 separate body makes body 32 in component "bin (3)"
shell "Shell1'''" thickness 10 removed faces 1 at (781.7342, 216.6667, 825) on bodies 32 in component "bin (3)"
sketch "Sketch57" plane through (-484.9325, 0, 0) normal (-1, 0, 0) x (0, -1, 0)
  line L0 (-100, 0) -> (-100, 25)
  line L1 (-100, 25) -> (-450, 25)
  line L2 (-450, 25) -> (-450, 800)
  line L3 (-450, 800) -> (-100, 800)
  line L4 (-100, 800) -> (-100, 25)
  line L5 (-100, 25) -> (-75, 25)
  line L6 (-75, 25) -> (-75, 825)
  line L7 (-75, 825) -> (-475, 825)
  line L8 (-475, 825) -> (-475, 0)
  line L9 (-475, 0) -> (-100, 0)
  line L10 (-450, 75) -> (-475, 75)
  line L11 (-475, 75) -> (-475, 100)
  line L12 (-475, 100) -> (-450, 100)
  line L13 (-450, 100) -> (-450, 75)
  dimension "d388" = 25
  dimension "d389" = 50
  constraint horizontal L10
  constraint vertical L11
  constraint horizontal L12
  constraint vertical L13
  constraint coincident L8 L11.end
  constraint coincident L2 L10.start
  measures "d388" distance of L10 L12
  measures "d389" distance of L1 L10
extrude "Extrude36" add sketch "Sketch57" against normal blind 1500 contours L2 L8 L10 L11 L12 L13 bodies 9 in component "bin case (1)"
sketch "Sketch58" plane through (0, 475, 0) normal (0, 1, 0) x (-1, 0, 0)
  line L0 (-1015.0675, 100) -> (-1015.0675, 825)
  line L1 (-1015.0675, 825) -> (-1040.0675, 825)
  line L2 (-1040.0675, 825) -> (-1040.0675, 0)
  line L3 (-1040.0675, 0) -> (484.9325, 0)
  line L4 (484.9325, 0) -> (484.9325, 825)
  line L5 (484.9325, 825) -> (459.9325, 825)
  line L6 (459.9325, 825) -> (459.9325, 100)
  line L7 (459.9325, 100) -> (109.9325, 100)
  line L8 (109.9325, 100) -> (109.9325, 825)
  line L9 (109.9325, 825) -> (84.9325, 825)
  line L10 (84.9325, 825) -> (84.9325, 100)
  line L11 (84.9325, 100) -> (-265.0675, 100)
  line L12 (-265.0675, 100) -> (-265.0675, 825)
  line L13 (-265.0675, 825) -> (-290.0675, 825)
  line L14 (-290.0675, 825) -> (-290.0675, 100)
  line L15 (-290.0675, 100) -> (-640.0675, 100)
  line L16 (-640.0675, 100) -> (-640.0675, 825)
  line L17 (-640.0675, 825) -> (-665.0675, 825)
  line L18 (-665.0675, 825) -> (-665.0675, 100)
  line L19 (-665.0675, 100) -> (-1015.0675, 100)
  line L20 (459.9325, 75) -> (459.9325, 25)
  line L21 (459.9325, 25) -> (109.9325, 25)
  line L22 (109.9325, 25) -> (109.9325, 75)
  line L23 (109.9325, 75) -> (459.9325, 75)
  line L24 (-1015.0675, 75) -> (-665.0675, 75)
  line L25 (-665.0675, 75) -> (-665.0675, 25)
  line L26 (-665.0675, 25) -> (-1015.0675, 25)
  line L27 (-1015.0675, 25) -> (-1015.0675, 75)
  line L28 (-290.0675, 75) -> (-290.0675, 25)
  line L29 (-290.0675, 25) -> (-640.0675, 25)
  line L30 (-640.0675, 25) -> (-640.0675, 75)
  line L31 (-640.0675, 75) -> (-290.0675, 75)
  line L32 (-265.0675, 75) -> (84.9325, 75)
  line L33 (84.9325, 75) -> (84.9325, 25)
  line L34 (84.9325, 25) -> (-265.0675, 25)
  line L35 (-265.0675, 25) -> (-265.0675, 75)
  line L36 (-1015.0675, 75) -> (-1040.0675, 75)
  line L37 (-1040.0675, 75) -> (-1040.0675, 100)
  line L38 (-1040.0675, 100) -> (-1015.0675, 100)
  line L39 (-1015.0675, 100) -> (-1015.0675, 75)
  line L40 (-665.0675, 100) -> (-640.0675, 100)
  line L41 (-640.0675, 100) -> (-640.0675, 75)
  line L42 (-640.0675, 75) -> (-665.0675, 75)
  line L43 (-665.0675, 75) -> (-665.0675, 100)
  line L44 (-290.0675, 100) -> (-265.0675, 100)
  line L45 (-265.0675, 100) -> (-265.0675, 75)
  line L46 (-265.0675, 75) -> (-290.0675, 75)
  line L47 (-290.0675, 75) -> (-290.0675, 100)
  line L48 (84.9325, 100) -> (109.9325, 100)
  line L49 (109.9325, 100) -> (109.9325, 75)
  line L50 (109.9325, 75) -> (84.9325, 75)
  line L51 (84.9325, 75) -> (84.9325, 100)
  line L52 (459.9325, 100) -> (484.9325, 100)
  line L53 (484.9325, 100) -> (484.9325, 75)
  line L54 (484.9325, 75) -> (459.9325, 75)
  line L55 (459.9325, 75) -> (459.9325, 100)
  dimension "d394" = 1500
  dimension "d395" = 0
  constraint horizontal L36
  constraint vertical L37
  constraint horizontal L38
  constraint vertical L39
  constraint coincident L2 L37.end
  constraint coincident L24.start L27.end
extrude "Extrude37" add sketch "Sketch58" against normal blind 400 contours L2 L36 L37 L38 L39 | L40 L41 L42 L43 | L44 L45 L46 L47 | L48 L49 L50 L51 | L4 L52 L53 L54 L55 bodies 9 in component "bin case (1)"
sketch "Sketch59" plane through (-484.9325, 0, 0) normal (-1, 0, 0) x (0, -1, 0)
  line L0 (-450, 100) -> (-450, 800)
  line L1 (-450, 800) -> (-100, 800)
  line L2 (-100, 800) -> (-100, 100)
  line L3 (-100, 100) -> (-450, 100)
  line L4 (-450, 75) -> (-100, 75)
  line L5 (-100, 75) -> (-100, 25)
  line L6 (-100, 25) -> (-75, 25)
  line L7 (-75, 25) -> (-75, 825)
  line L8 (-75, 825) -> (-475, 825)
  line L9 (-475, 825) -> (-475, 0)
  line L10 (-475, 0) -> (-100, 0)
  line L11 (-100, 0) -> (-100, 25)
  line L12 (-100, 25) -> (-450, 25)
  line L13 (-450, 25) -> (-450, 75)
  line L14 (-100, 100) -> (-75, 100)
  line L15 (-75, 100) -> (-75, 75)
  line L16 (-75, 75) -> (-100, 75)
  line L17 (-100, 75) -> (-100, 100)
  constraint horizontal L14
  constraint vertical L15
  constraint horizontal L16
  constraint vertical L17
  constraint coincident L7 L15.end
  constraint coincident L2.end L3.start
extrude "Extrude38" add sketch "Sketch59" against normal blind 1525 contours L7 L14 L15 L16 L17 bodies 9 in component "bin case (1)"
extrude "Extrude39" cut 1 faces at (998.3333, -445, 1066.6667) along direction (0, 1, 0) blind 25 on bodies 9 bodies 9 in component "bin case (1)"
sketch "Sketch60" plane through (0, 0, 825) normal (0, 0, 1) x (-1, 0, 0)
  line L0 (-640.0675, -475) -> (-640.0675, -100)
  line L1 (-640.0675, -100) -> (-290.0675, -100)
  line L2 (-290.0675, -100) -> (-290.0675, -475)
  line L3 (-290.0675, -475) -> (-265.0675, -475)
  line L4 (-265.0675, -475) -> (-265.0675, -100)
  line L5 (-265.0675, -100) -> (84.9325, -100)
  line L6 (84.9325, -100) -> (84.9325, -475)
  line L7 (84.9325, -475) -> (109.9325, -475)
  line L8 (109.9325, -475) -> (109.9325, -100)
  line L9 (109.9325, -100) -> (459.9325, -100)
  line L10 (459.9325, -100) -> (459.9325, -475)
  line L11 (459.9325, -475) -> (484.9325, -475)
  line L12 (484.9325, -475) -> (484.9325, -75)
  line L13 (484.9325, -75) -> (-1220.0675, -75)
  line L14 (-1220.0675, -75) -> (-1220.0675, -100)
  line L15 (-1220.0675, -100) -> (-1040.0675, -100)
  line L16 (-1040.0675, -100) -> (-1040.0675, -475)
  line L17 (-1040.0675, -475) -> (-1015.0675, -475)
  line L18 (-1015.0675, -475) -> (-1015.0675, -100)
  line L19 (-1015.0675, -100) -> (-665.0675, -100)
  line L20 (-665.0675, -100) -> (-665.0675, -475)
  line L21 (-665.0675, -475) -> (-640.0675, -475)
  line L22 (-1220.0675, -75) -> (-1040.0675, -75)
  line L23 (-1040.0675, -75) -> (-1040.0675, -87.5)
  line L24 (-1040.0675, -87.5) -> (-1220.0675, -87.5)
  line L25 (-1220.0675, -87.5) -> (-1220.0675, -75)
  dimension "d406" = 180
  constraint horizontal L22
  constraint vertical L23
  constraint horizontal L24
  constraint vertical L25
  constraint coincident L13.end L14.start
  measures "d406" distance of L23 L25
extrude "Extrude1'''''''''''" add sketch "Sketch60" along normal blind 150 separate body contours L13 L14 L22 L23 L24 L25 makes body 33 in component "limit"
extrude "Extrude2'''''''''" add 1 faces at (1220.0675, 79.1667, 875) along direction (1, 0, 0) blind 50 on bodies 33 bodies 33 in component "limit"
sketch "Sketch61" plane through (0, 0, 825) normal (0, 0, 1) x (-1, 0, 0)
  line L0 (-640.0675, -475) -> (-640.0675, -100)
  line L1 (-640.0675, -100) -> (-290.0675, -100)
  line L2 (-290.0675, -100) -> (-290.0675, -475)
  line L3 (-290.0675, -475) -> (-265.0675, -475)
  line L4 (-265.0675, -475) -> (-265.0675, -100)
  line L5 (-265.0675, -100) -> (84.9325, -100)
  line L6 (84.9325, -100) -> (84.9325, -475)
  line L7 (84.9325, -475) -> (109.9325, -475)
  line L8 (109.9325, -475) -> (109.9325, -100)
  line L9 (109.9325, -100) -> (459.9325, -100)
  line L10 (459.9325, -100) -> (459.9325, -475)
  line L11 (459.9325, -475) -> (484.9325, -475)
  line L12 (484.9325, -475) -> (484.9325, -75)
  line L13 (484.9325, -75) -> (-1220.0675, -75)
  line L14 (-1220.0675, -75) -> (-1220.0675, -100)
  line L15 (-1220.0675, -100) -> (-1040.0675, -100)
  line L16 (-1040.0675, -100) -> (-1040.0675, -475)
  line L17 (-1040.0675, -475) -> (-1015.0675, -475)
  line L18 (-1015.0675, -475) -> (-1015.0675, -100)
  line L19 (-1015.0675, -100) -> (-665.0675, -100)
  line L20 (-665.0675, -100) -> (-665.0675, -475)
  line L21 (-665.0675, -475) -> (-640.0675, -475)
  line L22 (-640.0675, -100) -> (-665.0675, -100)
  line L23 (-665.0675, -100) -> (-665.0675, -300)
  line L24 (-665.0675, -300) -> (-640.0675, -300)
  line L25 (-640.0675, -300) -> (-640.0675, -100)
  line L26 (-265.0675, -100) -> (-290.0675, -100)
  line L27 (-290.0675, -100) -> (-290.0675, -300)
  line L28 (-290.0675, -300) -> (-265.0675, -300)
  line L29 (-265.0675, -300) -> (-265.0675, -100)
  line L30 (109.9325, -100) -> (84.9325, -100)
  line L31 (84.9325, -100) -> (84.9325, -300)
  line L32 (84.9325, -300) -> (109.9325, -300)
  line L33 (109.9325, -300) -> (109.9325, -100)
  arc A0 (-640.0675, -100) -> (-665.0675, -100) centre (-652.5675, -90.625) ccw
  arc A1 (-265.0675, -100) -> (-290.0675, -100) centre (-277.5675, -90.625) ccw
  arc A2 (109.9325, -100) -> (84.9325, -100) centre (97.4325, -90.625) ccw
  dimension "d411" = 200
  dimension "d412" = 200
  dimension "d413" = 200
  constraint horizontal L22
  constraint vertical L23
  constraint horizontal L24
  constraint vertical L25
  constraint coincident L0.end L1.start
  constraint horizontal L26
  constraint vertical L27
  constraint horizontal L28
  constraint vertical L29
  constraint coincident L4.end L5.start
  constraint horizontal L30
  constraint vertical L31
  constraint horizontal L32
  constraint vertical L33
  constraint coincident L6 L31.end
  constraint coincident L8.end L9.start
  constraint tangent L13 A0
  constraint coincident L19.end L20.start
  constraint tangent L13 A1
  constraint tangent L13 A2
  measures "d411" distance of L0.end L24.end
  measures "d412" distance of L4.end L28.end
  measures "d413" distance of L30 L32
extrude "Extrude40" add sketch "Sketch61" along normal blind 50 contours L0 L20 L22 L23 L24 L25 | L22 A0 | L2 L4 L26 L27 L28 L29 | L26 A1 | L6 L8 L30 L31 L32 L33 | L30 A2 bodies 9 in component "bin case (1)"
extrude "Extrude41" cut 1 faces at (-459.5009, 263.1797, 891.6667) along direction (0.573576, -0.819152, 0) blind 100 on bodies 9 bodies 9 in component "bin case (1)"
extrude "Extrude42" cut 1 faces at (-436.286, 238.7425, 860.3333) along direction (-0.819152, -0.573576, 0) blind 10 on bodies 9 bodies 9 in component "bin case (1)"
loft "Loft1''''" add profiles "Sketch55", "Sketch56" section 1 contours L18 L19 L20 L26 L27 L28 L29 | L22 L23 L24 L25 section 2 contours L35 L53 L54 L55 | L35 L40 L53 L55 | L40 L42 L53 L55 | L29 L42 L53 L55 | L29 L52 L53 L55 separate body makes body 34 in component "bin (4)"
shell "Shell1''''" thickness 10 removed faces 1 at (781.7342, 216.6667, 825) on bodies 34 in component "bin (4)"
extrude "Extrude1''''''''''''" cut 1 faces at (785.0685, 446.6656, 825) along direction (0, 0, -1) blind 225 on bodies 34 bodies 34 in component "bin (4)"
extrude "Extrude2''''''''''" cut 1 faces at (895.0665, 110.0031, 675) along direction (0, 1, 0) blind 328.524 on bodies 34 bodies 34 in component "bin (4)"
extrude "Extrude3'''''" cut 1 faces at (785.0685, 439.9969, 750) along direction (0, -1, 0) blind 225 on bodies 34 bodies 34 in component "bin (4)"
sketch "Sketch62" plane through (-485, 0, 0) normal (-1, 0, 0) x (0, -1, 0)
  line L0 (180, 0) -> (180, 800)
  line L1 (180, 800) -> (155, 800)
  line L2 (155, 800) -> (155, 25)
  line L3 (155, 25) -> (-100, 25)
  line L4 (-100, 25) -> (-100, 0)
  line L5 (-100, 0) -> (180, 0)
  line L6 (155, 125) -> (180, 125)
  line L7 (180, 125) -> (180, 150)
  line L8 (180, 150) -> (155, 150)
  line L9 (155, 150) -> (155, 125)
  line L10 (155, 200) -> (180, 200)
  line L11 (180, 200) -> (180, 225)
  line L12 (180, 225) -> (155, 225)
  line L13 (155, 225) -> (155, 200)
  dimension "d426" = 25
  dimension "d427" = 25
  dimension "d428" = 100
  dimension "d429" = 50
  constraint horizontal L6
  constraint vertical L7
  constraint horizontal L8
  constraint vertical L9
  constraint coincident L2 L6.start
  constraint horizontal L10
  constraint vertical L11
  constraint horizontal L12
  constraint vertical L13
  constraint coincident L2 L10.start
  measures "d426" distance of L6.start L8.end
  measures "d427" distance of L10.start L12.end
  measures "d428" distance of L3 L6
  measures "d429" distance of L8 L10
extrude "Extrude43" add sketch "Sketch62" along normal blind 375 contours L0 L2 L6 L7 L8 L9 | L0 L2 L10 L11 L12 L13 bodies 9 in component "bin case (1)"
sketch "Sketch63" plane through (0, -155, 0) normal (0, 1, 0) x (-1, 0, 0)
  line L0 (250, 900) -> (250, 875)
  line L1 (250, 875) -> (460, 875)
  line L2 (460, 875) -> (460, 825)
  line L3 (460, 825) -> (-215, 825)
  line L4 (-215, 825) -> (-590, 825)
  line L5 (-590, 825) -> (-965, 825)
  line L6 (-965, 825) -> (-1015, 825)
  line L7 (-1015, 825) -> (-1015, 875)
  line L8 (-1015, 875) -> (160, 875)
  line L9 (160, 875) -> (160, 900)
  line L10 (160, 900) -> (-1040, 900)
  line L11 (-1040, 900) -> (-1040, 825)
  line L12 (-1040, 825) -> (-1220, 825)
  line L13 (-1220, 825) -> (-1250.0621, 808.2988)
  arc A0 (-1248.0189, 784.434) -> (-1250.0621, 808.2988) centre (-1265, 795) ccw
  line L14 (-1248.0189, 784.434) -> (-1220, 800)
  line L15 (-1220, 800) -> (-1040, 800)
  line L16 (-1040, 800) -> (-1040, 25)
  line L17 (-1040, 25) -> (-1015, 25)
  line L18 (-1015, 25) -> (-1015, 800)
  line L19 (-1015, 800) -> (-290, 800)
  line L20 (-290, 800) -> (-290, 25)
  line L21 (-290, 25) -> (-265, 25)
  line L22 (-265, 25) -> (-265, 800)
  line L23 (-265, 800) -> (460, 800)
  line L24 (460, 800) -> (460, 25)
  line L25 (460, 25) -> (485, 25)
  line L26 (485, 25) -> (485, 125)
  line L27 (485, 125) -> (860, 125)
  line L28 (860, 125) -> (860, 150)
  line L29 (860, 150) -> (485, 150)
  line L30 (485, 150) -> (485, 200)
  line L31 (485, 200) -> (860, 200)
  line L32 (860, 200) -> (860, 225)
  line L33 (860, 225) -> (485, 225)
  line L34 (485, 225) -> (485, 800)
  line L35 (485, 800) -> (486, 800)
  line L36 (486, 800) -> (518.7278, 783.3022)
  arc A1 (519.6212, 807.8463) -> (518.7278, 783.3022) centre (534.95, 795) ccw
  line L37 (519.6212, 807.8463) -> (486, 825)
  line L38 (486, 825) -> (485, 825)
  line L39 (485, 825) -> (485, 875)
  line L40 (485, 875) -> (485, 900)
  line L41 (485, 900) -> (250, 900)
  line L42 (860, 150) -> (835, 150)
  line L43 (835, 150) -> (835, 125)
  line L44 (835, 125) -> (860, 125)
  line L45 (860, 125) -> (860, 150)
  line L46 (860, 200) -> (835, 200)
  line L47 (835, 200) -> (835, 225)
  line L48 (835, 225) -> (860, 225)
  line L49 (860, 225) -> (860, 200)
  dimension "d432" = 25
  dimension "d433" = 25
  constraint horizontal L42
  constraint vertical L43
  constraint horizontal L44
  constraint vertical L45
  constraint coincident L27 L43.end
  constraint coincident L28.end L29.start
  constraint horizontal L46
  constraint vertical L47
  constraint horizontal L48
  constraint vertical L49
  constraint coincident L33 L47.end
  constraint coincident L31.end L32.start
  measures "d432" distance of L47 L49
  measures "d433" distance of L43 L45
extrude "Extrude44" add sketch "Sketch63" along normal blind 375 contours L31 L32 L33 L46 L47 L48 L49 | L27 L28 L29 L42 L43 L44 L45 bodies 9 in component "bin case (1)"